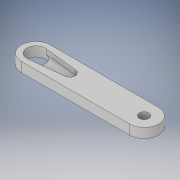
# Autodesk Inventor part: Stewart_ServoArm
Saved by Autodesk Inventor 2018.1 (Build 221171000, 171)
## iProperties
Created: 2017-11-13
Part Number: Stewart_ServoArm
Material: Generic
Document SubType Name: Modeling
Designer: sodie
Density: 1 g/cm^3
Appearance: Default
Author: sodie
Autodesk Inventor part; units mm, degrees
note: some values were not read from the file. Chosen so that the rebuilt part matches the saved one: sketch regions of "Extrusion2".
ref_plane "YZ Plane" through (0, 0, 0) normal (1, 0, 0) x (0, 1, 0)
ref_plane "XZ Plane" through (0, 0, 0) normal (0, 1, 0) x (-1, 0, 0)
ref_plane "XY Plane" through (0, 0, 0) normal (0, 0, 1) x (1, 0, 0)
sketch "Sketch1" plane through (0, 0, 0) normal (0, 1, 0) x (-1, 0, 0)
  circle A0 centre (0, 0) radius 3.75
  circle A1 centre (0, 0) radius 6
  circle A2 centre (-45, 0) radius 2
  circle A3 centre (-45, 0) radius 6
  line L0 (0, 6) -> (-45, 6)
  line L1 (0, -6) -> (-45, -6)
  dimension "d0" = 7.5
  dimension "d1" = 12
  dimension "d2" = 4
  dimension "d3" = 45
  dimension "d4" = 12
  constraints: 4 centre point, 4 end point, 4 point on circle, 3 coincident, 2 tangent, 1 horizontal alignment
  measures "d0" diameter of A0
  measures "d1" diameter of A1
  measures "d2" diameter of A2
  measures "d3" distance of point (0, 0) A2.centre
  measures "d4" diameter of A3
extrude "Extrusion2" add sketch "Sketch1" along normal blind 4
sketch "Sketch2" plane through (0, 4, 0) normal (0, 1, 0) x (1, 0, 0)
  arc A0 (14.3366, -2.2384) -> (14.3439, 2.2376) centre (14.108, 0) ccw
  circle A1 centre (0, 0) radius 3.75 projected
  arc A2 (0.7821, 3.6675) -> (2.5223, -2.775) centre (0, 0) ccw
  line L0 (0.7821, 3.6675) -> (14.3439, 2.2376)
  line L1 (14.3366, -2.2384) -> (0, -3.75)
  point P0 (2.5223, 2.775)
  dimension "d9" = 14.108
  dimension "d10" = 4.5
  dimension "d11" = 2.775
  dimension "d12" = 2.5223
  dimension "d13" = 5.55
  constraints: 6 point on circle, 4 end point, 2 centre point, 2 coincident, 1 horizontal alignment, 1 tangent, 3 other
  measures "d9" distance of point (0, 0) point (14.108, 0)
  measures "d10" diameter of A0
  measures "d11" vertical distance of point (0, 0) point (2.522, 2.775)
  measures "d12" horizontal distance of point (0, 0) point (2.522, 2.775)
  measures "d13" distance of A2.end point (2.522, 2.775)
extrude "Extrusion3" cut sketch "Sketch2" against normal blind 2 contours L1 A1 L0 A0
body "Solid2"
